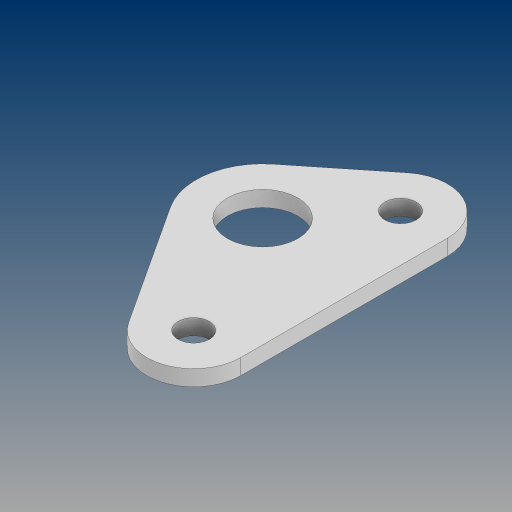
# Autodesk Inventor part: DragBarLinkage3 Bar2
Saved by Autodesk Inventor 2024.3 (Build 283343000, 343)
## iProperties
Created: 2024-07-08
Part Number: DragBarLinkage3 Bar2
Material: Generic
Document SubType Name: Modeling
Designer: Kenji
Density: 1 g/cm^3
Appearance: Default
Author: Kenji
Autodesk Inventor part; units mm, degrees
ref_plane "YZ Plane" through (0, 0, 0) normal (1, 0, 0) x (0, 1, 0)
ref_plane "XZ Plane" through (0, 0, 0) normal (0, 1, 0) x (-1, 0, 0)
ref_plane "XY Plane" through (0, 0, 0) normal (0, 0, 1) x (1, 0, 0)
sketch "Sketch1" plane through (0, 0, 0) normal (0, 1, 0) x (-1, 0, 0)
  line L0 (0, 0) -> (0, -83.82) construction
  circle A0 centre (0, -83.82) radius 6.35
  circle A1 centre (0, 0) radius 6.35
  circle A2 centre (25.4, -53.34) radius 14.2875
  line L1 (0, -83.82) -> (0, -53.34) construction
  circle A3 centre (25.4, -53.34) radius 26.9875 construction
  line L2 (0, -53.34) -> (25.4, -53.34) construction
  circle A4 centre (0, 0) radius 19.05 construction
  circle A5 centre (0, -83.82) radius 19.05 construction
  line L3 (-19.05, 0) -> (-19.05, -83.82)
  line L4 (42.2569, -74.4154) -> (11.899, -98.6967)
  line L5 (47.9861, -38.5687) -> (15.9432, 10.4268)
  arc A6 (42.2569, -74.4154) -> (47.9861, -38.5687) centre (25.4, -53.34) ccw
  arc A7 (15.9432, 10.4268) -> (-19.05, 0) centre (0, 0) ccw
  arc A8 (-19.05, -83.82) -> (11.899, -98.6967) centre (0, -83.82) ccw
  dimension "d0" = 83.82
  dimension "d1" = 12.7
  dimension "d2" = 12.7
  dimension "d4" = 28.575
  dimension "d5" = 30.48
  dimension "d6" = 12.7
  dimension "d7" = 25.4
  dimension "d8" = 12.7
  dimension "d9" = 12.7
  constraints: 12 end point, 12 point on circle, 10 tangent, 9 centre point, 3 coincident, 1 concentric, 1 horizontal, 1 point on line, 1 vertical
  measures "d0" distance of L0.start L0.end
  measures "d1" diameter of A0
  measures "d2" diameter of A1
  measures "d4" diameter of A2
  measures "d5" distance of L1.start L1.end
  measures "d6" radial gap between concentric circles of A2 A3
  measures "d7" distance of L1.end L2.end
  measures "d8" radial gap between concentric circles of A1 A4
  measures "d9" radial gap between concentric circles of A0 A5
extrude "Extrusion1" add sketch "Sketch1" along normal blind 6.35
body "Solid1"
